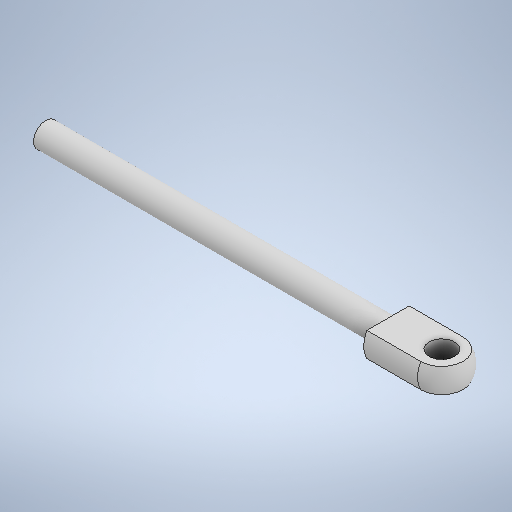
# Autodesk Inventor part: 21.2
Saved by Autodesk Inventor 2025.1 (Build 291241000, 241)
## iProperties
Created: 2024-09-13
Part Number: 21.2
Material: Generisch
Document SubType Name: Modeling
Designer: ffogue
Density: 1 g/cm^3
Appearance: Vorgabe
Author: ffogue
Autodesk Inventor part; units mm, degrees
ref_plane "YZ Plane" through (0, 0, 0) normal (1, 0, 0) x (0, 1, 0)
ref_plane "XY Plane" through (0, 0, 0) normal (0, 0, 1) x (1, 0, 0)
sketch "Sketch1" plane through (0, 0, 0) normal (0, 0, 1) x (1, 0, 0)
  line L0 (0, 0) -> (43, 0)
  arc A0 (43, 0) -> (40.5, 2.5) centre (40.5, 0) ccw
  line L1 (40.5, 2.5) -> (35, 2.5)
  line L2 (35, 2.5) -> (35, 1.25)
  line L3 (35, 1.25) -> (0, 1.25)
  line L4 (0, 1.25) -> (0, 0)
  point P0 (0, 0.625)
  dimension "d0" = 2.5
  dimension "d1" = 5.5
  dimension "d2" = 2.5
  dimension "d3" = 40.5
  constraints: 10 end point, 3 perpendicular, 2 point on circle, 1 centre point, 1 horizontal, 1 midpoint, 1 parallel, 1 point on line, 1 vertical alignment
  measures "d0" radius of A0
  measures "d1" distance of L1.start L1.end
  measures "d2" diameter of L3 L0
  measures "d3" horizontal distance of point (0, 0.625) A0.centre
revolve "Revolution1" add sketch "Sketch1" angle 360 about axis through (0, 0, 0) along (1, 0, 0)
ref_plane "Work Plane1" through (0, 5, 0) normal (0, 1, 0) x (-1, 0, 0)
sketch "Sketch2" plane through (0, 5, 0) normal (0, 1, 0) x (-1, 0, 0)
  arc A0 (-40.5, 2.5) -> (-40.5, -2.5) centre (-40.5, 0) ccw projected
  line L0 (-35, -1.25) -> (-35, 1.25) construction
  line L1 (-40.5, 2.5) -> (-40.5, -2.5) construction
  line L2 (-35, 2.5) -> (-35, -2.5) projected
  line L3 (-35, -1.25) -> (-42.6651, -1.25)
  line L4 (-35, 1.25) -> (-42.6651, 1.25)
  line L5 (-35, -2.5) -> (-40.5, -2.5) projected
  line L6 (-35, 2.5) -> (-40.5, 2.5) projected
  point P0 (0, 0)
  point P1 (-35, 0)
  dimension "d6" = 2.5
  dimension "d9" = 2.5
  dimension "d10" = 1.25
  constraints: 6 end point, 2 midpoint, 2 point on circle, 1 horizontal, 1 horizontal alignment, 1 parallel, 3 other
  measures "d6" distance of L0.start L0.end
  measures "d9" distance between parallel lines of L4 L3
  measures "d10" distance from line of point (-40.5, 0) L3
extrude "Extrusion2" cut sketch "Sketch2" against normal blind 10 contours L6 L2 L4 A0 | L3 L2 L5 A0
sketch "Sketch3" plane through (40.5, -2.1651, -1.25) normal (0, 0, -1) x (-1, 0, 0)
  arc A0 (0, 4.3301) -> (0, 0) centre (0, 2.1651) ccw projected
  point P0 (40.5, 2.1651)
  constraints: 1 coincident
hole "Hole1" at (40.5, 0, -1.25) direction (0, 0, 1) diameter 2.6 depth 2.5
equation "\"d10\" = 0.5 * d9"
body "Solid1"
